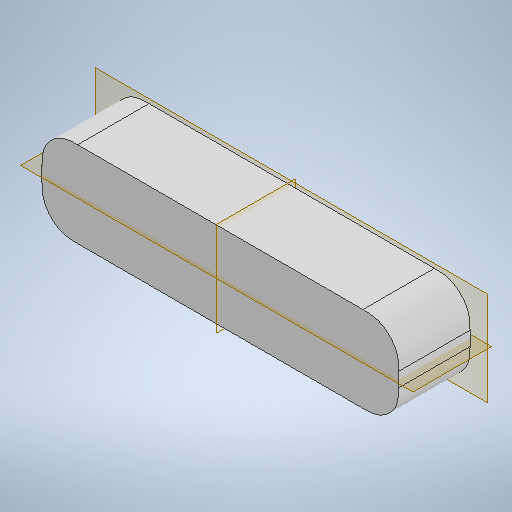
# Autodesk Inventor part: EjectorArm
Saved by Autodesk Inventor 2025.1 (Build 291241000, 241)
## iProperties
Created: 2025-02-22
Part Number: EjectorArm
Material: Generic
Document SubType Name: Modeling
Designer: 13156
Density: 1 g/cm^3
Appearance: Default
Author: 13156
Autodesk Inventor part; units mm, degrees
sketch "Sketch1" plane through (0, 0, 0) normal (0, 0, 1) x (1, 0, 0)
  line L0 (-16.5825, 1.7845) -> (-5.2923, 2.9472)
  line L1 (-5.2923, 2.9472) -> (-16.5825, 1.7845)
  arc A0 (-16.5825, 1.7845) -> (-16.5804, -1.9959) centre (-16.3889, -0.1056) ccw
  arc A1 (-16.5825, 1.7845) -> (-16.5804, -1.9959) centre (-16.3889, -0.1056) ccw
  line L2 (-5.2883, -3.1399) -> (-16.5804, -1.9959)
  line L3 (-16.5804, -1.9959) -> (-5.2883, -3.1399)
  line L4 (-5.2883, -3.1399) -> (-5.2889, -4.0963)
  line L5 (4.7111, -3.1398) -> (4.7111, -4.0963)
  line L6 (4.7111, -4.0963) -> (4.7111, -3.1398)
  line L7 (4.7111, -3.1398) -> (16.0026, -1.996)
  line L8 (4.7111, -3.1398) -> (16.0026, -1.996)
  line L9 (16.0048, 1.7845) -> (4.7152, 2.9472)
  arc A2 (16.0026, -1.996) -> (16.0048, 1.7845) centre (15.8111, -0.1056) ccw
  line L10 (16.0048, 1.7845) -> (4.7152, 2.9472)
  line L11 (4.7077, 3.9037) -> (4.7152, 2.9472)
  line L12 (-5.2923, 3.9037) -> (4.7077, 3.9037)
  line L13 (4.7077, 3.9037) -> (-5.2923, 3.9037)
  line L14 (-5.2923, 3.9037) -> (-5.2923, 2.9472)
  line L15 (4.7111, -4.0963) -> (-5.2889, -4.0963)
  line L16 (-5.2889, -4.0963) -> (4.7111, -4.0963)
  line L17 (-35, 0) -> (35, 0) projected
  line L18 (0, 8.4) -> (0, -8.4) projected
  line L19 (-25, 6) -> (25, 6)
  line L20 (25, 6) -> (25, -6)
  line L21 (25, -6) -> (-25, -6)
  line L22 (-25, -6) -> (-25, 6)
  point P0 (0, 0)
  point P1 (4.7111, -0.0963)
  point P2 (17.7111, -0.1067)
  point P3 (-18.2889, -0.1067)
  point P4 (-5.2886, -3.6181)
  dimension "d0" = 10
  dimension "d1" = 36
  dimension "d2" = 8
  dimension "d3" = 11.2902
  dimension "d4" = 1.1627
  dimension "d5" = 3.9037
  dimension "d6" = 16.3889
  dimension "d7" = 1.9
  dimension "d8" = 0.9565
  dimension "d9" = 0.9565
  dimension "d10" = 0.9565
  dimension "d11" = 0.9565
  dimension "d12" = 1.8903
  dimension "d13" = 5.2923
  dimension "d14" = 4.7111
  dimension "d15" = 5.2886
  dimension "d16" = 15.8111
  dimension "d17" = 50
  dimension "d18" = 12
  constraints: 42 end point, 12 equal length, 8 point on circle, 3 centre point, 2 horizontal, 2 perpendicular, 1 equal radius, 1 midpoint, 1 tangent, 2 other
  measures "d0" distance of L5.end L4.end
  measures "d1" distance of point (17.711, -0.107) point (-18.289, -0.107)
  measures "d2" distance between parallel lines of L15 L12
  measures "d3" horizontal distance of L0.start L0.end
  measures "d4" vertical distance of L0.start L0.end
  measures "d5" distance between parallel lines of L17 L12
  measures "d6" distance from line of L18 A1.centre
  measures "d7" radius of A2
  measures "d8" distance of L5.end L5.start
  measures "d9" distance of L4.end L2.start
  measures "d10" distance from line of L9.end L12
  measures "d11" distance of L0.end L12.start
  measures "d12" vertical distance of A0.centre L2.end
  measures "d13" distance from line of L18 L0.end
  measures "d14" distance from line of L18 L5.start
  measures "d15" distance from line of L18 point (-5.289, -3.618)
  measures "d16" distance from line of L18 A2.centre
  measures "d17" distance of L19.start L19.end
  measures "d18" distance between parallel lines of L21 L19
extrude "Extrusion2" add sketch "Sketch1" along normal blind 10 contours A0 L17 L22 L19 L18 L12 L14 L0 | A0 L2 L4 L15 L18 L21 L22 L17 | L18 L19 L20 L17 A2 L9 L11 L12 | L17 L20 L21 L18 L15 L5 L7 A2
sketch "Sketch2" plane through (0, 0, 10) normal (0, 0, 1) x (1, 0, 0)
  line L0 (-25, 6) -> (-25, -6) projected
  line L1 (-25, -6) -> (25, -6) projected
  line L2 (-25, 6) -> (25, 6)
  line L3 (25, 6) -> (25, -6)
  line L4 (25, -6) -> (-25, -6)
  line L5 (-25, -6) -> (-25, 6)
  point P0 (0, 0)
  constraints: 8 end point, 2 parallel, 1 horizontal, 1 perpendicular
extrude "Extrusion3" add sketch "Sketch2" against normal blind 7.5
sketch "Sketch4" plane through (0, 0, 2.5) normal (0, 0, -1) x (-1, 0, 0)
  line L0 (5.2923, 3.9037) -> (-4.7077, 3.9037) projected
  line L1 (-4.7111, -4.0963) -> (5.2889, -4.0963) projected
  line L2 (-4.7077, 3.9037) -> (5.2889, 3.9037)
  line L3 (5.2889, 3.9037) -> (5.2889, -4.0963)
  line L4 (5.2889, -4.0963) -> (-4.7077, -4.0963)
  line L5 (-4.7077, -4.0963) -> (-4.7077, 3.9037)
  point P0 (0, 0)
  constraints: 8 end point, 2 parallel, 1 horizontal, 1 perpendicular
extrude "Extrusion4" cut sketch "Sketch4" against normal blind 1
fillet "Fillet1" radius 5 4 edges at (25, 6, 5) (-25, 6, 5) (-25, -6, 5) (25, -6, 5) curvature continuous yes
body "Solid2"
